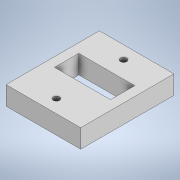
# Autodesk Inventor part: AdaptadorSensorInductivoV4
Saved by Autodesk Inventor 2020.3 (Build 243373000, 373)
## iProperties
Created: 2020-09-23
Part Number: AdaptadorSensorInductivoV4
Material: Generic
Document SubType Name: Modeling
Designer: mifer
Density: 1 g/cm^3
Appearance: Default
Author: mifer
## iProperties of the stored document _3DPrint.ipt
Created: 2020-09-23
Part Number: _3DPrint
Material: Generic
Document SubType Name: Modeling
Designer: mifer
Density: 1 g/cm^3
Appearance: Default
Author: mifer
Autodesk Inventor part; units mm, degrees
ref_plane "YZ Plane" through (0, 0, 0) normal (1, 0, 0) x (0, 1, 0)
ref_plane "XZ Plane" through (0, 0, 0) normal (0, 1, 0) x (-1, 0, 0)
ref_plane "XY Plane" through (0, 0, 0) normal (0, 0, 1) x (1, 0, 0)
sketch "Sketch1" plane through (0, 0, 0) normal (0, 1, 0) x (-1, 0, 0)
  line L0 (0, 0) -> (40, 0)
  line L1 (40, 0) -> (40, -50)
  line L2 (40, -50) -> (0, -50)
  line L3 (0, -50) -> (0, 0)
  line L4 (40, 0) -> (0, 0)
  line L5 (0, 0) -> (0, -18)
  line L6 (5, -18) -> (35, -18)
  line L7 (40, -18) -> (40, 0)
  line L8 (35, -18) -> (5, -18)
  line L9 (0, -18) -> (0, -37)
  line L10 (5, -37) -> (35, -37)
  line L11 (40, -37) -> (40, -18)
  circle A0 centre (20, -7) radius 1.7
  circle A1 centre (20, -43) radius 1.7
  line L12 (20, -18) -> (35, -18)
  line L13 (35, -18) -> (35, -37)
  line L14 (35, -37) -> (20, -37)
  line L15 (20, -37) -> (5, -37)
  line L16 (5, -37) -> (5, -18)
  line L17 (5, -18) -> (20, -18)
  line L18 (35, -21) -> (5, -21)
  line L19 (5, -21) -> (5, -34)
  line L20 (5, -34) -> (35, -34)
  line L21 (35, -34) -> (35, -21)
  dimension "d0" = 40
  dimension "d1" = 50
  dimension "d2" = 3.4
  dimension "d3" = 3.4
  dimension "d6" = 19
  constraints: 44 end point, 10 parallel, 6 horizontal, 6 perpendicular, 4 point on line, 2 centre point, 1 midpoint
  measures "d0" distance of L1.end L2.end
  measures "d1" distance of L0.end L1.end
  measures "d2" diameter of A0
  measures "d3" diameter of A1
  measures "d6" distance between parallel lines of L10 L6
extrude "Extrusion1" add sketch "Sketch1" along normal blind 10 contours L0 L1 L2 L3 | L6 L13 L18 L16 | L20 L13 L10 L16
body "Solid1"
